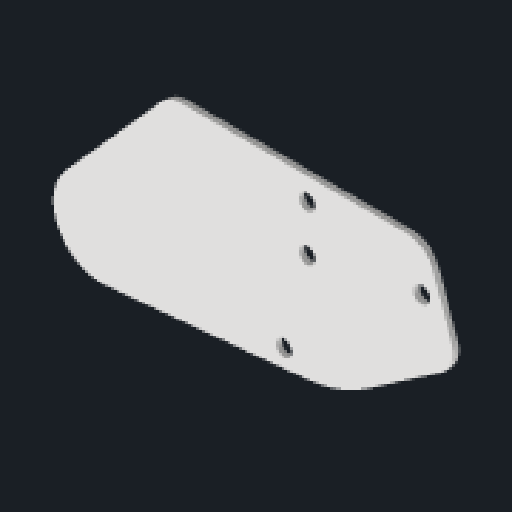
# Autodesk Inventor part: neil
Saved by Autodesk Inventor 2024.2 (Build 282272000, 272)
## iProperties
Created: 2024-01-18
Part Number: neil
Material: Generic
Document SubType Name: Modeling
Designer: reima
Density: 1 g/cm^3
Appearance: Default
Author: reima
Autodesk Inventor part; units mm, degrees
ref_plane "YZ Plane" through (0, 0, 0) normal (1, 0, 0) x (0, 1, 0)
ref_plane "XZ Plane" through (0, 0, 0) normal (0, 1, 0) x (-1, 0, 0)
ref_plane "XY Plane" through (0, 0, 0) normal (0, 0, 1) x (1, 0, 0)
sketch "Sketch1" plane through (0, 0, 0) normal (0, 0, 1) x (1, 0, 0)
  circle A0 centre (53.3707, -52.9691) radius 2.2352
  arc A1 (-7.0885, -40.7359) -> (4.0322, -62.6709) centre (2.7723, -49.5231) ccw
  arc A2 (94.5267, -13.6218) -> (87.3345, -8.5191) centre (87.3345, -16.1391) ccw
  line L0 (25.0369, -8.5191) -> (87.3345, -8.5191)
  arc A3 (96.8127, -37.2153) -> (99.7022, -28.4091) centre (92.51, -30.9263) ccw
  line L1 (99.7022, -28.4091) -> (94.5267, -13.6218)
  arc A4 (59.2846, -57.3763) -> (76.4278, -51.1618) centre (55.7999, -21.0109) ccw
  arc A5 (25.0369, -8.5191) -> (19.348, -11.0695) centre (25.0369, -16.1391) ccw
  circle A6 centre (59.7207, -27.5691) radius 2.2352
  circle A7 centre (91.4707, -21.2191) radius 2.2352
  circle A8 centre (59.7207, -14.8691) radius 2.2352
  line L2 (76.4278, -51.1618) -> (96.8127, -37.2153)
  line L3 (19.348, -11.0695) -> (-7.0885, -40.7359)
  line L4 (4.0322, -62.6709) -> (59.2846, -57.3763)
  point P0 (0, 0)
  point P1 (19.348, -11.0695)
  point P2 (-7.0885, -40.7359)
  point P3 (4.0322, -62.6709)
  point P4 (59.2846, -57.3763)
  point P5 (76.4278, -51.1618)
  point P6 (94.5267, -13.6218)
  point P7 (87.3345, -8.5191)
  constraints: 10 end point, 10 point on circle, 9 centre point
extrude "Extrusion1" add sketch "Sketch1" along normal blind 1.5875
body "Solid1"
